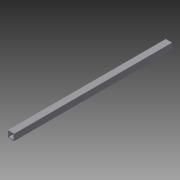
# Autodesk Inventor part: backlong
Saved by Autodesk Inventor 2013 SP2 (Build 170200200, 200)
## iProperties
Created: 2015-01-07
Part Number: backlong
Material: Generic
Document SubType Name: Modeling
Designer: darkb_000
Density: 1 g/cm^3
Author: darkb_000
Autodesk Inventor part; units mm, degrees
ref_plane "YZ Plane" through (0, 0, 0) normal (1, 0, 0) x (0, 1, 0)
ref_plane "XZ Plane" through (0, 0, 0) normal (0, 1, 0) x (-1, 0, 0)
ref_plane "XY Plane" through (0, 0, 0) normal (0, 0, 1) x (1, 0, 0)
sketch "Sketch1" plane through (0, 0, 0) normal (0, 0, 1) x (1, 0, 0)
  line L0 (0, 0) -> (-25.4, 0) projected
  line L1 (-25.4, -711.2) -> (-25.4, 0) projected
  line L2 (-25.4, 0) -> (0, 0)
  line L3 (0, 0) -> (0, -25.4)
  line L4 (0, -25.4) -> (-25.4, -25.4)
  line L5 (-25.4, -25.4) -> (-25.4, 0)
  dimension "d0" = 25.4
  dimension "d1" = 25.4
  constraints: 8 end point, 2 parallel, 1 horizontal, 1 perpendicular
  measures "d0" distance of L3.end L4.end
  measures "d1" distance of L2.end L3.end
ref_plane "Work Plane1" through (-25.4, -711.2, 635) normal (0, 0, -1) x (0, 1, 0)
extrude "Extrusion1" add sketch "Sketch1" along normal up to surface (635 mm away)
sketch "Sketch2" plane through (-25.4, 0, 635) normal (0, 0, 1) x (1, 0, 0)
  line L0 (0, 0) -> (3.175, 0)
  line L1 (3.175, 0) -> (3.175, -3.175)
  line L2 (3.175, -3.175) -> (0, -3.175)
  line L3 (0, -3.175) -> (0, 0)
  line L4 (25.4, -25.4) -> (22.225, -25.4)
  line L5 (22.225, -25.4) -> (22.225, -22.225)
  line L6 (22.225, -22.225) -> (25.4, -22.225)
  line L7 (25.4, -22.225) -> (25.4, -25.4)
  line L8 (22.225, -22.225) -> (3.175, -22.225)
  line L9 (3.175, -22.225) -> (3.175, -3.175)
  line L10 (3.175, -3.175) -> (22.225, -3.175)
  line L11 (22.225, -3.175) -> (22.225, -22.225)
  dimension "d4" = 3.175
  dimension "d5" = 3.175
  dimension "d6" = 3.175
  dimension "d7" = 3.175
  constraints: 24 end point, 6 parallel, 3 horizontal, 3 perpendicular
  measures "d4" distance of L1.end L2.end
  measures "d5" distance of L0.end L1.end
  measures "d6" distance of L5.end L6.end
  measures "d7" distance of L4.end L5.end
extrude "Extrusion2" cut sketch "Sketch2" against normal through all contours L10 L11 L8 L9
body "Solid1"
